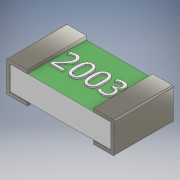
# Autodesk Inventor part: 21-1001
Saved by Autodesk Inventor 2018 (Build 220112000, 112)
## iProperties
Created: 2019-09-21
Part Number: 21-1001
Material: Copper
Document SubType Name: Modeling
Designer: Bradley
Density: 8.94 g/cm^3
Appearance: Smooth - White
Author: Bradley
Autodesk Inventor part; units mm, degrees
ref_plane "YZ Plane" through (0, 0, 0) normal (1, 0, 0) x (0, 1, 0)
ref_plane "XZ Plane" through (0, 0, 0) normal (0, 1, 0) x (-1, 0, 0)
ref_plane "XY Plane" through (0, 0, 0) normal (0, 0, 1) x (1, 0, 0)
sketch "Sketch1" plane through (0, 0, 0) normal (0, 1, 0) x (-1, 0, 0)
  line L0 (0.725, 0.175) -> (-0.725, 0.175)
  line L1 (-0.725, 0.175) -> (-0.725, -0.175)
  line L2 (-0.725, -0.175) -> (0.725, -0.175)
  line L3 (0.725, -0.175) -> (0.725, 0.175)
  line L4 (0.475, 0.175) -> (0.475, 0.225)
  line L5 (0.475, 0.225) -> (0.775, 0.225)
  line L6 (0.775, 0.225) -> (0.775, -0.225)
  line L7 (0.775, -0.225) -> (0.475, -0.225)
  line L8 (0.475, -0.225) -> (0.475, -0.175)
  line L9 (-0.475, 0.175) -> (-0.475, 0.225)
  line L10 (-0.475, 0.225) -> (-0.775, 0.225)
  line L11 (-0.775, 0.225) -> (-0.775, -0.225)
  line L12 (-0.775, -0.225) -> (-0.475, -0.225)
  line L13 (-0.475, -0.175) -> (-0.475, -0.225)
  line L14 (0.475, 0.175) -> (-0.475, 0.175)
  point P0 (0, 0)
  point P1 (0, 0.175)
  point P2 (0.725, 0)
  dimension "d0" = 1.55
  dimension "d1" = 0.05
  dimension "d2" = 0.05
  dimension "d3" = 0.45
  dimension "d4" = 0.3
  constraints: 30 end point, 12 point on line, 7 perpendicular, 3 collinear, 3 midpoint, 2 parallel, 1 horizontal, 1 horizontal alignment, 1 vertical, 1 vertical alignment
  measures "d0" distance between parallel lines of L11 L6
  measures "d1" distance of L7.end L8.end
  measures "d2" distance between parallel lines of L6 L3
  measures "d3" distance of L5.end L6.end
  measures "d4" distance of L6.end L7.end
extrude "Extrusion1" add sketch "Sketch1" along normal mid plane 0.85 contours L0 L4 L5 L6 L7 L8 L2 L3 | L0 L1 L2 L13 L12 L11 L10 L9
extrude "Extrusion2" add sketch "Sketch1" along normal mid plane 0.84 contours L3 L2 L1 L0
sketch "Sketch2" plane through (-0.475, -0.42, 0.175) normal (0, 0, 1) x (1, 0, 0)
  line L0 (0, 0) -> (0, 0.84) projected
  line L1 (0.95, 0) -> (0, 0) projected
  line L2 (0.95, 0) -> (0.95, 0.84) projected
  line L3 (0, 0.84) -> (0.95, 0.84) projected
  line L4 (0, 0.42) -> (0.95, 0.42) construction
  line L5 (0.2316, 0.27) -> (0.0466, 0.27)
  line L6 (0.0466, 0.27) -> (0.0466, 0.3125)
  spline S0 degree 2 poles (0.0466, 0.3125) (0.0666, 0.3313) (0.1021, 0.366) (0.1191, 0.3847) knots 0 0 0 1 2 2 2
  spline S1 degree 2 poles (0.1191, 0.3847) (0.1534, 0.4224) (0.1784, 0.4676) (0.1784, 0.4917) knots 0 0 0 1 2 2 2
  spline S2 degree 2 poles (0.1784, 0.4917) (0.1784, 0.5044) (0.1706, 0.5233) (0.1636, 0.5294) knots 0 0 0 1 2 2 2
  spline S3 degree 2 poles (0.1636, 0.5294) (0.1565, 0.5355) (0.138, 0.5416) (0.1269, 0.5416) knots 0 0 0 1 2 2 2
  spline S4 degree 2 poles (0.1269, 0.5416) (0.1162, 0.5416) (0.0943, 0.5362) (0.0843, 0.5321) knots 0 0 0 1 2 2 2
  spline S5 degree 2 poles (0.0843, 0.5321) (0.0758, 0.5287) (0.06, 0.5189) (0.0551, 0.5155) knots 0 0 0 1 2 2 2
  line L7 (0.0551, 0.5155) -> (0.053, 0.5155)
  line L8 (0.053, 0.5155) -> (0.053, 0.5583)
  spline S6 degree 2 poles (0.053, 0.5583) (0.0654, 0.5644) (0.1098, 0.5763) (0.1298, 0.5763) knots 0 0 0 1 2 2 2
  spline S7 degree 2 poles (0.1298, 0.5763) (0.1718, 0.5763) (0.2192, 0.5318) (0.2192, 0.4939) knots 0 0 0 1 2 2 2
  spline S8 degree 2 poles (0.2192, 0.4939) (0.2192, 0.4762) (0.211, 0.4465) (0.2037, 0.4339) knots 0 0 0 1 2 2 2
  spline S9 degree 2 poles (0.2037, 0.4339) (0.1964, 0.4207) (0.1752, 0.395) (0.1636, 0.3826) knots 0 0 0 1 2 2 2
  spline S10 degree 2 poles (0.1636, 0.3826) (0.1446, 0.3619) (0.0982, 0.3176) (0.0843, 0.3048) knots 0 0 0 1 2 2 2
  line L9 (0.0843, 0.3048) -> (0.2316, 0.3048)
  line L10 (0.2316, 0.3048) -> (0.2316, 0.27)
  spline S11 degree 2 poles (0.4585, 0.42) (0.4585, 0.3393) (0.4115, 0.2637) (0.3627, 0.2637) knots 0 0 0 1 2 2 2
  spline S12 degree 2 poles (0.3627, 0.2637) (0.3131, 0.2637) (0.2667, 0.3407) (0.2667, 0.4198) knots 0 0 0 1 2 2 2
  spline S13 degree 2 poles (0.2667, 0.4198) (0.2667, 0.501) (0.3136, 0.5761) (0.3627, 0.5761) knots 0 0 0 1 2 2 2
  spline S14 degree 2 poles (0.3627, 0.5761) (0.412, 0.5761) (0.4585, 0.4983) (0.4585, 0.42) knots 0 0 0 1 2 2 2
  spline S15 degree 2 poles (0.4069, 0.3286) (0.4128, 0.3434) (0.4176, 0.3891) (0.4176, 0.42) knots 0 0 0 1 2 2 2
  spline S16 degree 2 poles (0.4176, 0.42) (0.4176, 0.4509) (0.4128, 0.4963) (0.4067, 0.5117) knots 0 0 0 1 2 2 2
  spline S17 degree 2 poles (0.4067, 0.5117) (0.4006, 0.527) (0.3795, 0.5428) (0.3627, 0.5428) knots 0 0 0 1 2 2 2
  spline S18 degree 2 poles (0.3627, 0.5428) (0.3459, 0.5428) (0.3243, 0.527) (0.3179, 0.5112) knots 0 0 0 1 2 2 2
  spline S19 degree 2 poles (0.3179, 0.5112) (0.3119, 0.4959) (0.3075, 0.4492) (0.3075, 0.4198) knots 0 0 0 1 2 2 2
  spline S20 degree 2 poles (0.3075, 0.4198) (0.3075, 0.3882) (0.3114, 0.3459) (0.3177, 0.3293) knots 0 0 0 1 2 2 2
  spline S21 degree 2 poles (0.3177, 0.3293) (0.3235, 0.3138) (0.3452, 0.297) (0.3627, 0.297) knots 0 0 0 1 2 2 2
  spline S22 degree 2 poles (0.3627, 0.297) (0.3792, 0.297) (0.4009, 0.3128) (0.4069, 0.3286) knots 0 0 0 1 2 2 2
  spline S23 degree 2 poles (0.6836, 0.42) (0.6836, 0.3393) (0.6367, 0.2637) (0.5878, 0.2637) knots 0 0 0 1 2 2 2
  spline S24 degree 2 poles (0.5878, 0.2637) (0.5382, 0.2637) (0.4918, 0.3407) (0.4918, 0.4198) knots 0 0 0 1 2 2 2
  spline S25 degree 2 poles (0.4918, 0.4198) (0.4918, 0.501) (0.5387, 0.5761) (0.5878, 0.5761) knots 0 0 0 1 2 2 2
  spline S26 degree 2 poles (0.5878, 0.5761) (0.6372, 0.5761) (0.6836, 0.4983) (0.6836, 0.42) knots 0 0 0 1 2 2 2
  spline S27 degree 2 poles (0.6321, 0.3286) (0.6379, 0.3434) (0.6427, 0.3891) (0.6427, 0.42) knots 0 0 0 1 2 2 2
  spline S28 degree 2 poles (0.6427, 0.42) (0.6427, 0.4509) (0.6379, 0.4963) (0.6318, 0.5117) knots 0 0 0 1 2 2 2
  spline S29 degree 2 poles (0.6318, 0.5117) (0.6257, 0.527) (0.6046, 0.5428) (0.5878, 0.5428) knots 0 0 0 1 2 2 2
  spline S30 degree 2 poles (0.5878, 0.5428) (0.571, 0.5428) (0.5494, 0.527) (0.5431, 0.5112) knots 0 0 0 1 2 2 2
  spline S31 degree 2 poles (0.5431, 0.5112) (0.537, 0.4959) (0.5326, 0.4492) (0.5326, 0.4198) knots 0 0 0 1 2 2 2
  spline S32 degree 2 poles (0.5326, 0.4198) (0.5326, 0.3882) (0.5365, 0.3459) (0.5428, 0.3293) knots 0 0 0 1 2 2 2
  spline S33 degree 2 poles (0.5428, 0.3293) (0.5487, 0.3138) (0.5703, 0.297) (0.5878, 0.297) knots 0 0 0 1 2 2 2
  spline S34 degree 2 poles (0.5878, 0.297) (0.6043, 0.297) (0.626, 0.3128) (0.6321, 0.3286) knots 0 0 0 1 2 2 2
  spline S35 degree 2 poles (0.803, 0.5416) (0.792, 0.5416) (0.7704, 0.5362) (0.7599, 0.5321) knots 0 0 0 1 2 2 2
  spline S36 degree 2 poles (0.7599, 0.5321) (0.7502, 0.5279) (0.7359, 0.5192) (0.7303, 0.5153) knots 0 0 0 1 2 2 2
  line L11 (0.7303, 0.5153) -> (0.7278, 0.5153)
  line L12 (0.7278, 0.5153) -> (0.7278, 0.5578)
  spline S37 degree 2 poles (0.7278, 0.5578) (0.741, 0.5649) (0.7859, 0.5763) (0.8061, 0.5763) knots 0 0 0 1 2 2 2
  spline S38 degree 2 poles (0.8061, 0.5763) (0.8265, 0.5763) (0.8569, 0.5681) (0.8693, 0.5593) knots 0 0 0 1 2 2 2
  spline S39 degree 2 poles (0.8693, 0.5593) (0.8825, 0.5498) (0.8961, 0.5224) (0.8961, 0.5039) knots 0 0 0 1 2 2 2
  spline S40 degree 2 poles (0.8961, 0.5039) (0.8961, 0.4791) (0.8635, 0.4416) (0.8406, 0.4368) knots 0 0 0 1 2 2 2
  line L13 (0.8406, 0.4368) -> (0.8406, 0.4339)
  spline S41 degree 2 poles (0.8406, 0.4339) (0.8501, 0.4319) (0.8718, 0.4232) (0.881, 0.4144) knots 0 0 0 1 2 2 2
  spline S42 degree 2 poles (0.881, 0.4144) (0.8902, 0.4059) (0.9019, 0.3787) (0.9019, 0.359) knots 0 0 0 1 2 2 2
  spline S43 degree 2 poles (0.9019, 0.359) (0.9019, 0.3388) (0.888, 0.3045) (0.8754, 0.2914) knots 0 0 0 1 2 2 2
  spline S44 degree 2 poles (0.8754, 0.2914) (0.8623, 0.2778) (0.8251, 0.2637) (0.8015, 0.2637) knots 0 0 0 1 2 2 2
  spline S45 degree 2 poles (0.8015, 0.2637) (0.7789, 0.2637) (0.7346, 0.2746) (0.7196, 0.2822) knots 0 0 0 1 2 2 2
  line L14 (0.7196, 0.2822) -> (0.7196, 0.3247)
  line L15 (0.7196, 0.3247) -> (0.7225, 0.3247)
  spline S46 degree 2 poles (0.7225, 0.3247) (0.7351, 0.3155) (0.7779, 0.2984) (0.7991, 0.2984) knots 0 0 0 1 2 2 2
  spline S47 degree 2 poles (0.7991, 0.2984) (0.8115, 0.2984) (0.8363, 0.3062) (0.8445, 0.3152) knots 0 0 0 1 2 2 2
  spline S48 degree 2 poles (0.8445, 0.3152) (0.8526, 0.3242) (0.8611, 0.3456) (0.8611, 0.3619) knots 0 0 0 1 2 2 2
  spline S49 degree 2 poles (0.8611, 0.3619) (0.8611, 0.3782) (0.8516, 0.3993) (0.8431, 0.4054) knots 0 0 0 1 2 2 2
  spline S50 degree 2 poles (0.8431, 0.4054) (0.8346, 0.4115) (0.8115, 0.4161) (0.7979, 0.4161) knots 0 0 0 1 2 2 2
  line L16 (0.7979, 0.4161) -> (0.7808, 0.4161)
  line L17 (0.7808, 0.4161) -> (0.7808, 0.4494)
  line L18 (0.7808, 0.4494) -> (0.7942, 0.4494)
  spline S51 degree 2 poles (0.7942, 0.4494) (0.8212, 0.4494) (0.8552, 0.4752) (0.8552, 0.4997) knots 0 0 0 1 2 2 2
  spline S52 degree 2 poles (0.8552, 0.4997) (0.8552, 0.5112) (0.8465, 0.5275) (0.8394, 0.5323) knots 0 0 0 1 2 2 2
  spline S53 degree 2 poles (0.8394, 0.5323) (0.8319, 0.5374) (0.8134, 0.5416) (0.803, 0.5416) knots 0 0 0 1 2 2 2
  point P0 (0.475, 0.42)
  constraints: 2 end point, 2 midpoint, 1 horizontal
extrude "Extrusion3" add sketch "Sketch2" along normal blind 0.02 contours L5 L6 S0 S1 S2 S3 S4 S5 L7 L8 S6 S7 S8 S9 S10 L9 L10 | S11 S12 S13 S14 | S23 S24 S25 S26 | S35 S36 L11 L12 S37 S38 S39 S40 L13 S41 S42 S43 S44 S45 L14 L15 S46 S47 S48 S49 S50 L16 L17 L18 S51 S52 S53
fillet "Fillet1" radius 0.02 4 edges at (-0.775, 0, 0.225) (-0.775, 0, -0.225) (0.775, 0, 0.225) (0.775, 0, -0.225)
equation "\"d2\" = d1"
body "Solid1"
